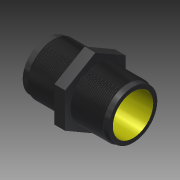
# Autodesk Inventor part: banjo nipple
Saved by Autodesk Inventor 2013 SP2 (Build 170200200, 200)
## iProperties
Created: 2014-07-09
Part Number: banjo nipple
Material: GFRP
Document SubType Name: Modeling
Designer: mrister
Density: 1.75 g/cm^3
Description: HEX NIPPLE, 1", (banjo NIP100SH)
Engineer: mrister
Author: mrister
Autodesk Inventor part; units mm, degrees
ref_plane "YZ Plane" through (0, 0, 0) normal (1, 0, 0) x (0, 1, 0)
ref_plane "XZ Plane" through (0, 0, 0) normal (0, 1, 0) x (-1, 0, 0)
ref_plane "XY Plane" through (0, 0, 0) normal (0, 0, 1) x (1, 0, 0)
sketch "Sketch1" plane through (0, 0, 0) normal (0, 0, 1) x (1, 0, 0)
  line L0 (-25.4, 11.9062) -> (25.4, 11.9063)
  line L1 (25.4, 11.9063) -> (25.4, 14.2875)
  line L2 (25.4, 14.2875) -> (-25.4, 14.2875)
  line L3 (-25.4, 14.2875) -> (-25.4, 11.9062)
  line L4 (0, 11.9062) -> (0, 0) construction
  line L5 (-35.56, 0) -> (35.56, 0) projected
  dimension "d0" = 50.8
  dimension "d2" = 11.9062
  dimension "d3" = 14.2875
  constraints: 10 end point, 2 perpendicular, 1 horizontal, 1 midpoint, 1 parallel, 1 vertical
  measures "d0" distance of L0.start L0.end
  measures "d2" distance of L4.start L4.end
  measures "d3" distance from line of L4.end L2
revolve "Revolution1" add sketch "Sketch1" angle 360 about axis through (-10, 0, 0) along (1, 0, 0)
sketch "Sketch2" plane through (0, 0, 0) normal (0, 0, 1) x (1, 0, 0)
  line L0 (32.9829, 14.2875) -> (33.7766, 14.2875)
  line L1 (33.7766, 14.2875) -> (33.3797, 15.0812)
  line L2 (33.3797, 15.0812) -> (32.9829, 14.2875)
  line L3 (33.3797, 15.0812) -> (33.3797, 14.2875) construction
  line L4 (-25.4, 14.2875) -> (25.4, 14.2875) construction
  point P0 (0, 0)
  dimension "d5" = 0.7937
  dimension "d8" = 0.7937
  constraints: 8 end point, 1 collinear, 1 horizontal, 1 midpoint, 1 vertical
  measures "d5" distance of L0.start L0.end
  measures "d8" distance of L1.end L3.end
coil "Coil1" sketch "Sketch2" operation add axis through (-10, 0, 0) along (-1, 0, 0) pitch 1.0583 turns 60 hand right
sketch "Sketch3" plane through (0, 0, 0) normal (0, 0, 1) x (1, 0, 0)
  line L0 (-43.8846, 22.5783) -> (-22.225, 22.5783)
  line L1 (-22.225, 22.5783) -> (-22.225, 14.2875)
  line L2 (-22.225, 14.2875) -> (-43.8846, 14.2875)
  line L3 (-43.8846, 14.2875) -> (-43.8846, 22.5783)
  line L4 (22.225, 22.5783) -> (43.8846, 22.5783)
  line L5 (43.8846, 22.5783) -> (43.8846, 14.2875)
  line L6 (43.8846, 14.2875) -> (22.225, 14.2875)
  line L7 (22.225, 14.2875) -> (22.225, 22.5783)
  line L8 (-61.4385, 0) -> (61.4385, 0) projected
  line L9 (-30.5171, 14.2875) -> (-29.7234, 14.2875) projected
  point P0 (0, 0)
  dimension "d17" = 8.2908
  dimension "d19" = 21.6596
  dimension "d20" = 44.45
  dimension "d21" = 22.225
  constraints: 16 end point, 4 collinear, 4 parallel, 2 horizontal, 2 perpendicular
  measures "d17" distance of L2.end L0.start
  measures "d19" distance of L0.start L0.end
  measures "d20" distance between parallel lines of L7 L1
  measures "d21" distance from line of point (0, 0) L7
revolve "Revolution2" cut sketch "Sketch3" angle 360 about axis through (-10, 0, 0) along (1, 0, 0)
sketch "Sketch4" plane through (0, 0, 0) normal (1, 0, 0) x (0, 1, 0)
  line L0 (-20.6222, 0) -> (-10.3111, 17.8594)
  line L1 (-10.3111, 17.8594) -> (10.3111, 17.8594)
  line L2 (10.3111, 17.8594) -> (20.6222, 0)
  line L3 (20.6222, 0) -> (10.3111, -17.8594)
  line L4 (10.3111, -17.8594) -> (-10.3111, -17.8594)
  line L5 (-10.3111, -17.8594) -> (-20.6222, 0)
  circle A0 centre (0, 0) radius 11.9063 projected
  dimension "d23" = 35.7188
  constraints: 12 end point, 1 coincident, 1 horizontal, 13 other
  measures "d23" distance between parallel lines of L3 L0
extrude "Extrusion1" add sketch "Sketch4" along normal mid plane 6.35
equation "\"d21\" = 0.5 * d20"
body "Solid1"
